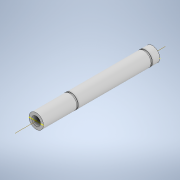
# Autodesk Inventor part: Shaft_potentiometer
Saved by Autodesk Inventor 2022 (Build 260153000, 153)
## iProperties
Created: 2022-04-28
Part Number: Shaft_potentiometer
Material: Generic
Document SubType Name: Sheet Metal
Designer: Malaika Din Hashmi
Density: 1 g/cm^3
Sheet Metal Rule: Default
Appearance: Default
Author: Malaika Din Hashmi
Autodesk Inventor part; units mm, degrees
ref_plane "YZ Plane" through (0, 0, 0) normal (1, 0, 0) x (0, 1, 0)
ref_plane "XZ Plane" through (0, 0, 0) normal (0, 1, 0) x (-1, 0, 0)
ref_plane "XY Plane" through (0, 0, 0) normal (0, 0, 1) x (1, 0, 0)
sketch "Sketch2" plane through (0, 0, 0) normal (0, 0, 1) x (1, 0, 0)
  circle A0 centre (0, 0) radius 5
  dimension "d0" = 10
  constraints: 1 centre point, 1 coincident
  measures "d0" diameter of A0
extrude "Extrusion1" add sketch "Sketch2" against normal blind 80
sketch "Sketch3" plane through (0, 0, 0) normal (0, 1, 0) x (-1, 0, 0)
  line L0 (-5, -80) -> (5, -80) projected
  line L1 (5, 0) -> (-5, 0) projected
  point P0 (0, 0)
sketch "Sketch4" plane through (0, 0, 0) normal (0, 1, 0) x (-1, 0, 0)
  line L0 (-5, 0) -> (-5, -80) projected
  line L1 (-5, -75) -> (-4.6, -75)
  line L2 (-4.6, -75) -> (-4.6, -74)
  line L3 (-4.6, -74) -> (-5, -74)
  line L4 (-5, -74) -> (-5, -75)
  line L5 (-5, -80) -> (5, -80) projected
  line L6 (0, -96) -> (0, 16) projected
  point P0 (0, 0)
  point P1 (-5, -74)
  dimension "d3" = 5
  dimension "d4" = 1
  dimension "d5" = 0.4
  constraints: 8 end point, 2 parallel, 1 horizontal, 1 perpendicular, 1 point on line
  measures "d3" distance between parallel lines of L1 L5
  measures "d4" distance of L1.end L2.end
  measures "d5" distance of L2.end L3.end
revolve "Revolution1" cut sketch "Sketch4" angle 360 about axis through (0, 0, 0) along (0, 0, 1)
sketch "Sketch5" plane through (0, 0, 0) normal (0, 1, 0) x (-1, 0, 0)
  line L0 (-5, 0) -> (-5, -74) projected
  line L1 (-5, -24) -> (-4.6, -24)
  line L2 (-4.6, -24) -> (-4.6, -23)
  line L3 (-4.6, -23) -> (-5, -23)
  line L4 (-5, -23) -> (-5, -24)
  line L5 (5, -74) -> (-5, -74) projected
  line L6 (0, -96) -> (0, 16) projected
  point P0 (0, 0)
  point P1 (-5, -23)
  dimension "d7" = 50
  dimension "d8" = 1
  dimension "d9" = 0.4
  constraints: 8 end point, 2 parallel, 1 horizontal, 1 perpendicular, 1 point on line
  measures "d7" distance between parallel lines of L5 L1
  measures "d8" distance of L1.end L2.end
  measures "d9" distance of L2.end L3.end
revolve "Revolution2" cut sketch "Sketch5" angle 360 about axis through (0, 0, 0) along (0, 0, 1)
sketch "Sketch7" plane through (0, 0, 0) normal (0, 0, 1) x (1, 0, 0)
  circle A0 centre (0, 0) radius 3
  dimension "d11" = 6
  constraints: 1 centre point, 1 coincident
  measures "d11" diameter of A0
extrude "Extrusion2" cut sketch "Sketch7" against normal blind 10
equation "\"BendRadius\" = Thickness"
equation "\"BendReliefWidth\" = Thickness"
equation "\"BendReliefDepth\" = 0.5 * Thickness"
equation "\"CornerReliefSize\" = 4 * Thickness"
equation "\"MinimumRemnant\" = 2 * Thickness"
equation "\"TransitionRadius\" = BendRadius"
equation "\"JacobiRadiusSize\" = BendRadius"
equation "\"GapSize\" = Thickness"
equation "\"Thickness\" = 3.048"
body "Solid1"
